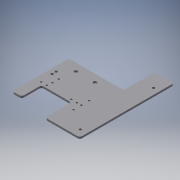
# Autodesk Inventor part: Part1
Saved by Autodesk Inventor 2016 (Build 200138000, 138)
## iProperties
Created: 2017-06-06
Part Number: Part1
Material: Generic
Document SubType Name: Modeling
Designer: m228540
Density: 1 g/cm^3
Appearance: Default
Author: m228540
Autodesk Inventor part; units mm, degrees
ref_plane "YZ Plane" through (0, 0, 0) normal (1, 0, 0) x (0, 1, 0)
ref_plane "XZ Plane" through (0, 0, 0) normal (0, 1, 0) x (-1, 0, 0)
ref_plane "XY Plane" through (0, 0, 0) normal (0, 0, 1) x (1, 0, 0)
ref_plane "Work Plane1" through (678.6266, 4, 0) normal (0, 0, 1) x (1, 0, 0)
sketch "Sketch1" plane through (678.6266, 4, 0) normal (0, 0, 1) x (1, 0, 0)
  line L0 (-6.4274, -1046.8384) -> (-66.4274, -1046.8384)
  line L1 (-116.4274, -1346.8384) -> (-6.4274, -1346.8384)
  line L2 (-6.4274, -1346.8384) -> (-6.4274, -1046.8384)
  line L3 (-116.4274, -1263.8384) -> (-211.4274, -1263.8384)
  line L4 (-211.4274, -1263.8384) -> (-211.4274, -1326.8384)
  line L5 (-211.4274, -1326.8384) -> (-241.4274, -1326.8384)
  line L6 (-241.4274, -1326.8384) -> (-241.4274, -1146.8384)
  line L7 (-116.4274, -1263.8384) -> (-116.4274, -1346.8384)
  line L8 (-241.4274, -1146.8384) -> (-66.4274, -1146.8384)
  line L9 (-66.4274, -1146.8384) -> (-66.4274, -1046.8384)
  point P0 (-678.6266, -4)
  dimension "d0" = 110
  dimension "d4" = 95
  dimension "d5" = 63
  dimension "d6" = 30
  dimension "d7" = 180
  dimension "d10" = 300
  dimension "d15" = 100
  constraints: 20 end point, 6 perpendicular, 2 horizontal, 2 parallel
  measures "d0" distance of L1.start L1.end
  measures "d4" distance of L3.start L3.end
  measures "d5" distance of L3.end L4.end
  measures "d6" distance of L4.end L5.end
  measures "d7" distance of L5.end L6.end
  measures "d10" distance of L1.end L0.start
  measures "d15" distance of L8.end L0.end
extrude "Extrusion1" add sketch "Sketch1" along normal blind 6
fillet "Fillet1" radius 7 10 edges at (612.1992, -1042.8384, 3) (672.1992, -1042.8384, 3) (437.1992, -1142.8384, 3) (437.1992, -1322.8384, 3) (467.1992, -1322.8384, 3) (467.1992, -1259.8384, 3) (562.1992, -1259.8384, 3) (562.1992, -1342.8384, 3) (672.1992, -1342.8384, 3) (612.1992, -1142.8384, 3)
sketch "Sketch2" plane through (678.6266, 4, 6) normal (0, 0, 1) x (1, 0, 0)
  circle A0 centre (-226.4274, -1296.8384) radius 4
  circle A1 centre (-226.4274, -1236.8384) radius 4
  circle A2 centre (-226.4274, -1176.8384) radius 4
  line L0 (-234.4274, -1326.8384) -> (-218.4274, -1326.8384) projected
  line L1 (-226.4274, -1326.8384) -> (-226.4274, -1296.8384) construction
  line L2 (-226.4274, -1296.8384) -> (-226.4274, -1236.8384) construction
  line L3 (-226.4274, -1236.8384) -> (-226.4274, -1176.8384) construction
  line L4 (-241.4274, -1153.8384) -> (-241.4274, -1319.8384) projected
  line L5 (-241.4274, -1236.8384) -> (-226.4274, -1236.8384) construction
  line L6 (-13.4274, -1046.8384) -> (-59.4274, -1046.8384) projected
  line L7 (-66.4274, -1053.8384) -> (-66.4274, -1139.8384) projected
  point P0 (-678.6266, -4)
  dimension "d17" = 8
  dimension "d18" = 60
  dimension "d19" = 60
  dimension "d27" = 30
  constraints: 8 end point, 3 centre point, 2 collinear, 2 equal radius, 2 midpoint, 1 perpendicular
  measures "d17" diameter of A0
  measures "d18" distance of L2.end L3.end
  measures "d19" distance of L1.end L2.end
  measures "d27" distance of L1.start L1.end
sketch "Sketch3" plane through (678.6266, 4, 6) normal (0, 0, 1) x (1, 0, 0)
  circle A0 centre (-193.7546, -1171.4413) radius 5.5 projected
  circle A1 centre (-133.7546, -1171.4413) radius 5.5 projected
  point P0 (-678.6266, -4)
extrude "Extrusion3" cut sketch "Sketch3" against normal through all
sketch "Sketch4" plane through (678.6266, 4, 6) normal (0, 0, 1) x (1, 0, 0)
  circle A0 centre (-25.4274, -1092.8384) radius 4 projected
  circle A1 centre (-27.4274, -1323.8384) radius 4 projected
  circle A2 centre (-225.4274, -1215.8384) radius 4 projected
  circle A3 centre (-225.4274, -1202.8384) radius 4 projected
  point P0 (-678.6266, -4)
extrude "Extrusion4" cut sketch "Sketch4" against normal through all
sketch "Sketch5" plane through (678.6266, 4, 6) normal (0, 0, 1) x (1, 0, 0)
  circle A0 centre (-92.7546, -1280.4413) radius 3 projected
  circle A1 centre (-92.7546, -1255.4413) radius 3 projected
  circle A2 centre (-92.7546, -1230.4413) radius 3 projected
  circle A3 centre (-106.7546, -1255.4413) radius 3 projected
  circle A4 centre (-124.7546, -1255.4413) radius 3 projected
  circle A5 centre (-202.7546, -1255.4413) radius 3 projected
  circle A6 centre (-220.7546, -1255.4413) radius 3 projected
  circle A7 centre (-198.7546, -1239.4413) radius 3 projected
  circle A8 centre (-198.7546, -1219.4413) radius 3 projected
  point P0 (-678.6266, -4)
extrude "Extrusion5" cut sketch "Sketch5" against normal through all
body "Solid1"
